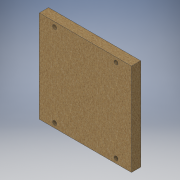
# Autodesk Inventor part: AkkuHaltBoden
Saved by Autodesk Inventor 2017 SP1 (Build 210196100, 196)
## iProperties
Part Number: AkkuHaltBoden
Material: Generisch
Document SubType Name: Modeling
Designer: Alex
Density: 1 g/cm^3
Appearance: Vorgabe
Author: Alex
Autodesk Inventor part; units mm, degrees
ref_plane "YZ Plane" through (0, 0, 0) normal (1, 0, 0) x (0, 1, 0)
ref_plane "XZ Plane" through (0, 0, 0) normal (0, 1, 0) x (-1, 0, 0)
ref_plane "XY Plane" through (0, 0, 0) normal (0, 0, 1) x (1, 0, 0)
sketch "Skizze1" plane through (0, 0, 0) normal (0, 1, 0) x (-1, 0, 0)
  line L0 (0, 0) -> (60, 0)
  line L1 (60, 0) -> (60, -60)
  line L2 (60, -60) -> (0, -60)
  line L3 (0, -60) -> (0, 0)
  dimension "d0" = 60
  dimension "d1" = 60
  constraints: 8 end point, 2 parallel, 1 horizontal, 1 perpendicular
  measures "d0" distance of L1.end L2.end
  measures "d1" distance of L0.end L1.end
extrude "Extrusion1" add sketch "Skizze1" along normal blind 6
sketch "m" plane through (0, 6, 0) normal (0, 1, 0) x (1, 0, 0)
  line L0 (-60, 0) -> (0, 0) projected
  line L1 (-60, 60) -> (-60, 0) projected
  line L2 (0, 0) -> (0, 60) projected
  line L3 (0, 60) -> (-60, 60) projected
  point P0 (-50, 3)
  point P1 (-10, 3)
  point P2 (-50, 57)
  point P3 (-10, 57)
  dimension "d4" = 3
  dimension "d5" = 10
  dimension "d6" = 10
  dimension "d7" = 3
  constraints: 2 horizontal alignment, 2 vertical alignment
  measures "d4" distance from line of L0 point (-50, 3)
  measures "d5" distance from line of point (-50, 3) L1
  measures "d6" distance from line of L2 point (-10, 3)
  measures "d7" distance from line of L3 point (-50, 57)
hole "Bohrung1" at (-50, 6, -3) at (-10, 6, -3) at (-50, 6, -57) at (-10, 6, -57) direction (0, -1, 0) diameter 2.5 depth 10 tip angle 118
chamfer "Fase1" distance 1 angle 45 4 edges at (-10, 6, -58.25) (-50, 6, -58.25) (-10, 6, -4.25) (-50, 6, -4.25)
